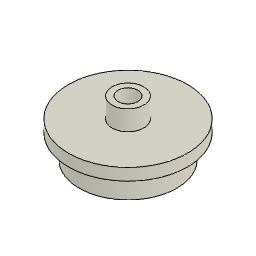
Traffic Light Diffuser v5 (Autodesk Fusion 360 design; units mm, degrees)
Autodesk Fusion 360 part; units mm, degrees
sketch "Sketch1" plane through (0, 0, 0) normal (0, 0, 1) x (1, 0, 0)
  circle A0 centre (0, 0) radius 12.3
  circle A1 centre (0, 0) radius 2.5
  circle A2 centre (0, 0) radius 4
  circle A3 centre (0, 0) radius 15
  dimension "d1" = 24.6
  dimension "led_diam" = 5
  dimension "d3" = 8
  dimension "d4" = 30
  constraint coincident A0.centre A1.centre
  constraint concentric A0 A1
  constraint concentric A0 A2
  constraint concentric A2 A3
  measures "d1" diameter of A0
  measures "led_diam" diameter of A1
  measures "d3" diameter of A2
  measures "d4" diameter of A3
extrude "Extrude1" add sketch "Sketch1" along normal blind 6 contours A0 | A1 | A2
extrude "Extrude2" add sketch "Sketch1" along normal blind 3 from surface at 6 contours A0 | A1 | A2 | A3
extrude "Extrude4" add sketch "Sketch1" along normal blind 5 from surface at 9 contours A2
equation "d3 = led_diam + 3 mm"
equation "diffuser_thick = 6 mm"
equation "light_offset = diffuser_thick"
equation "support_thick = 3 mm"
equation "d13 = diffuser_thick + support_thick"
